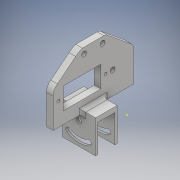
# Autodesk Inventor part: czesc glowna chwytaka
Saved by Autodesk Inventor 2017.2 (Build 212233000, 233)
## iProperties
Created: 2017-06-02
Part Number: czesc glowna chwytaka
Material: Ogólny
Document SubType Name: Modeling
Designer: magic
Density: 1 g/cm^3
Appearance: Domyślna
Author: magic
## iProperties of the stored document czesc glowna chwytaka _Drukowanie 3D.ipt
Created: 2017-06-02
Part Number: czesc glowna chwytaka _Drukowanie 3D
Material: Ogólny
Document SubType Name: Modeling
Designer: magic
Density: 1 g/cm^3
Appearance: Domyślna
Author: magic
Autodesk Inventor part; units mm, degrees
ref_plane "YZ Plane" through (0, 0, 0) normal (1, 0, 0) x (0, 1, 0)
ref_plane "XZ Plane" through (0, 0, 0) normal (0, 1, 0) x (-1, 0, 0)
ref_plane "XY Plane" through (0, 0, 0) normal (0, 0, 1) x (1, 0, 0)
sketch "Szkic1" plane through (0, 0, 0) normal (1, 0, 0) x (0, 1, 0)
  line L0 (0, 1.0111) -> (0, -17.7395)
  line L1 (0, -17.7395) -> (-48.7346, -17.7395)
  line L2 (-48.7346, -17.7395) -> (-48.7346, 0.2105)
  arc A0 (-46.1212, 5.2996) -> (-48.7346, 0.2105) centre (-42.4729, 0.2105) ccw
  line L3 (-46.1212, 5.2996) -> (-35.0263, 14.1821)
  arc A1 (-31.0007, 16.5663) -> (-35.0263, 14.1821) centre (-26.6278, 4.5922) ccw
  arc A2 (-15.4691, 15.5487) -> (-18, 16.5663) centre (-18, 12.9101) ccw
  arc A3 (0, 1.0111) -> (-1.3971, 3.9699) centre (-3.8316, 1.0111) ccw
  line L4 (-15.8982, 15.9018) -> (-1.3971, 3.9699)
  line L5 (-18, 16.5663) -> (-31.0007, 16.5663)
  circle A4 centre (-18.8067, 13.002) radius 1.5007
  circle A5 centre (-30, 13.0039) radius 1.4888
  circle A6 centre (-45.4922, -4) radius 0.9
  circle A7 centre (-12.7873, -3.975) radius 1.5
  circle A8 centre (-16.9979, -3.975) radius 0.9
  line L6 (-19.7721, 2.5223) -> (-19.7721, -10.4698)
  line L7 (-19.7721, -10.4698) -> (-42.6386, -10.4698)
  line L8 (-42.6386, -10.4698) -> (-42.6386, 2.5223)
  line L9 (-42.6386, 2.5223) -> (-19.7721, 2.5223)
  point P0 (0, 0)
  point P1 (0, -22.6354)
  dimension "d0" = 1.8
  dimension "d1" = 3
  dimension "d2" = 1.8
  constraints: 20 end point, 9 centre point, 9 point on circle, 4 perpendicular, 3 tangent, 2 horizontal, 2 vertical, 1 point on line
  measures "d0" diameter of A6
  measures "d1" diameter of A7
  measures "d2" diameter of A8
extrude "Wyciągnięcie proste1" add sketch "Szkic1" along normal blind 4 contours L0 L1 L2 A0 L3 A1 L5 A2 L4 A3
sketch "Szkic2" plane through (4, 0, 0) normal (1, 0, 0) x (0, 0, -1)
  line L0 (-16.5663, -18) -> (-16.5663, -31.0007) projected
  line L1 (-16.5663, -24.5004) -> (42, -24.5004)
  line L2 (16, -18.0004) -> (36, -18.0004)
  line L3 (36, -18.0004) -> (36, -31.0004)
  line L4 (36, -31.0004) -> (16, -31.0004)
  line L5 (16, -31.0004) -> (16, -18.0004)
  point P0 (0, 0)
  dimension "d5" = 20
  dimension "d6" = 13
  constraints: 10 end point, 2 horizontal, 2 parallel, 1 midpoint, 1 perpendicular, 1 other
  measures "d5" distance of L3.end L4.end
  measures "d6" distance of L2.end L3.end
extrude "Wyciągnięcie proste2" add sketch "Szkic2" against normal blind 12
sketch "Szkic3" plane through (-8, 0, 0) normal (-1, 0, 0) x (0, 0, 1)
  line L0 (-17.7395, -18.0004) -> (-16, -18.0004) projected
  line L1 (-36, -31.0004) -> (-17.7395, -31.0004) projected
  line L2 (-16, -18.0004) -> (-36, -18.0004)
  line L3 (-36, -18.0004) -> (-36, -31.0004)
  line L4 (-36, -31.0004) -> (-16, -31.0004)
  line L5 (-16, -31.0004) -> (-16, -18.0004)
  point P0 (0, 0)
  constraints: 8 end point, 2 parallel, 1 horizontal, 1 perpendicular
extrude "Wyciągnięcie proste3" add sketch "Szkic3" against normal blind 20
sketch "Szkic4" plane through (-8, -31.0004, -36) normal (0, 0, -1) x (-1, 0, 0)
  point P0 (-8, 31.0004)
sketch "Szkic5" plane through (-8, 0, 0) normal (-1, 0, 0) x (0, 0, 1)
  line L0 (-36, -18.0004) -> (-36, -31.0004) projected
  line L1 (-36, -29.6794) -> (-19, -29.6794)
  line L2 (-19, -29.6794) -> (-19, -19.3214)
  line L3 (-19, -19.3214) -> (-36, -19.3214)
  line L4 (-36, -19.3214) -> (-36, -29.6794)
  line L5 (-16, -31.0004) -> (-16, -18.0004) projected
  line L6 (-16, -24.5004) -> (-39.2975, -24.5004)
  point P0 (0, 0)
  constraints: 10 end point, 2 horizontal, 2 parallel, 1 midpoint, 1 perpendicular, 1 point on line, 1 other
extrude "Wyciągnięcie proste4" cut sketch "Szkic5" against normal blind 20
fillet "Zaokrąglenie1" radius 2 8 edges at (0, -31.0004, -16.8697) (0, -24.5004, -16) (0, -18.0004, -16.8697) (2, -18.0004, -17.7395) (4, -18.0004, -16.8697) (4, -24.5004, -16) (4, -31.0004, -16.8697) (2, -31.0004, -17.7395)
sketch "Szkic6" plane through (-8, -18.0004, -16) normal (0, 1, 0) x (1, 0, 0)
  line L0 (20, 20) -> (0, 20) projected
  line L1 (10, 20) -> (10, -8)
  circle A0 centre (10, 6.4693) radius 1.55
  arc A1 (15.9953, 14.4545) -> (4.2067, 14.6022) centre (10, 6.4693) ccw
  arc A2 (17.6193, 17.0025) -> (1.6495, 16.4327) centre (10, 6.4693) ccw
  arc A3 (15.9953, 14.4545) -> (17.6193, 17.0025) centre (16.7323, 15.7763) ccw
  arc A4 (1.6495, 16.4327) -> (4.2067, 14.6022) centre (3.2422, 15.9562) ccw
  line L2 (15.8971, 14.5272) -> (16.0005, 14.4516)
  line L3 (1.7865, 16.546) -> (1.6196, 16.3179)
  point P0 (8, -16)
  dimension "d14" = 3.1
  dimension "d17" = 26
  constraints: 12 point on circle, 6 end point, 5 centre point, 3 tangent, 2 coincident, 1 midpoint, 1 perpendicular, 1 point on line, 1 vertical
  measures "d14" diameter of A0
  measures "d17" diameter of A2
extrude "Wyciągnięcie proste5" cut sketch "Szkic6" against normal blind 20 contours A0 L1 | L1 A0
sketch "Szkic7" plane through (-8, -18.0004, -16) normal (0, 1, 0) x (1, 0, 0)
  line L0 (0, 20) -> (20, 20) projected
  line L1 (10, 20) -> (10, -4.2283)
  line L2 (20, 20) -> (20, 0) projected
  circle A0 centre (10, 4) radius 11
  circle A1 centre (10, 4) radius 14.025
  arc A2 (15.2148, 13.6853) -> (17.0707, 16.1122) centre (15.9483, 15.0475) ccw
  arc A3 (2.7167, 15.9856) -> (3.9993, 13.2191) centre (3.5134, 14.6744) ccw
  point P0 (8, -16)
  dimension "d18" = 10
  dimension "d19" = 22
  dimension "d20" = 28.05
  constraints: 8 point on circle, 4 centre point, 2 end point, 2 tangent, 1 coincident, 1 midpoint, 1 point on line, 1 vertical
  measures "d18" distance between parallel lines of L1 L2
  measures "d19" diameter of A0
  measures "d20" diameter of A1
extrude "Wyciągnięcie proste6" cut sketch "Szkic7" against normal blind 20 contours A1 A2 A0 L1 | L1 A0 A3 A1
